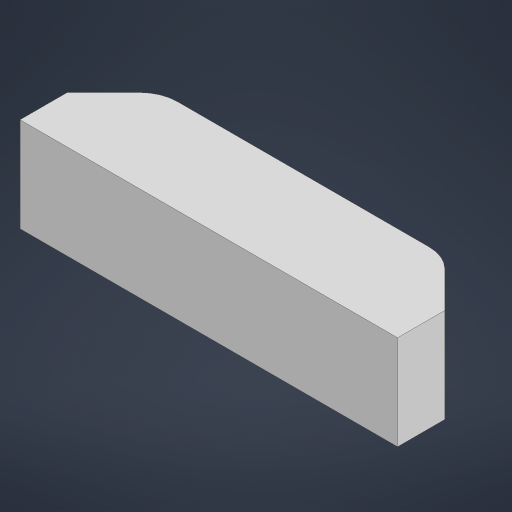
# Autodesk Inventor part: steal_glide_plate
Saved by Autodesk Inventor 2024 (Build 280153000, 153)
## iProperties
Created: 2023-05-24
Part Number: steal_glide_plate
Material: Generic
Document SubType Name: Modeling
Designer: aasmu
Density: 1 g/cm^3
Appearance: Default
Author: aasmu
Autodesk Inventor part; units mm, degrees
ref_plane "YZ Plane" through (0, 0, 0) normal (1, 0, 0) x (0, 1, 0)
ref_plane "XZ Plane" through (0, 0, 0) normal (0, 1, 0) x (-1, 0, 0)
ref_plane "XY Plane" through (0, 0, 0) normal (0, 0, 1) x (1, 0, 0)
sketch "Sketch1" plane through (0, 0, 0) normal (0, 1, 0) x (-1, 0, 0)
  line L0 (0, 0) -> (0, -2.5)
  line L1 (0, -2.5) -> (2.5, -5)
  line L2 (2.5, -5) -> (17.5, -5)
  line L3 (17.5, -5) -> (20, -2.5)
  line L4 (20, -2.5) -> (20, 0)
  line L5 (20, 0) -> (0, 0)
  point P0 (20, -1.25)
  dimension "d0" = 45
  dimension "d1" = 45
  dimension "d2" = 5
  dimension "d3" = 20
  dimension "d4" = 2.5
  constraints: 12 end point, 2 horizontal, 2 parallel, 1 midpoint, 1 vertical
  measures "d0" angle of L1 L0
  measures "d1" angle of L2 L3
  measures "d2" distance between parallel lines of L2 L5
  measures "d3" distance from line of L0 point (20, -1.25)
  measures "d4" distance of L0.start L0.end
extrude "Extrusion1" add sketch "Sketch1" along normal blind 5
fillet "Fillet1" radius 2 2 edges at (-2.5, 2.5, -5) (-17.5, 2.5, -5)
equation "\"d2\" = glide_plate_height"
equation "\"d3\" = glide_plate_length"
equation "\"d4\" = 0.5 * d2"
equation "\"d5\" = glide_plate_width"
equation "\"glide_plate_height\" = 5"
equation "\"glide_plate_length\" = 20"
equation "\"glide_plate_width\" = 5"
body "Solid1"
